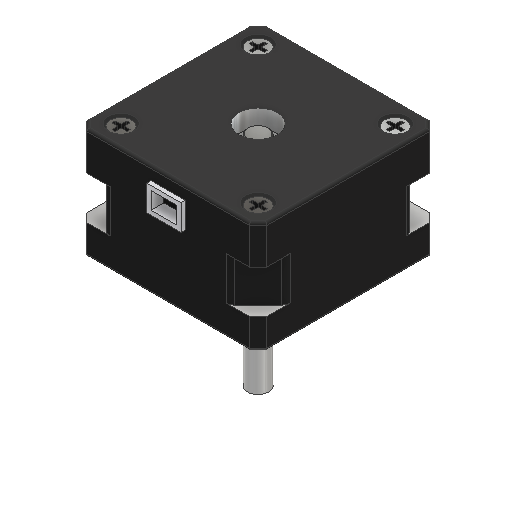
# Autodesk Inventor part: COTS_E3D_NEMA17_Pancake_Stepper_Extruder
Saved by Autodesk Inventor 2026.1 (Build 301233000, 233)
## iProperties
Created: 2016-01-19
Part Number: COTS_E3D_NEMA17_Pancake_Stepper_Extruder
Material: Ogólny
Document SubType Name: Modeling
Designer: Andrzej
Density: 1 g/cm^3
Appearance: Kauczuk - czarny
Mass: 82.3413 g
Surface Area: 122.845 cm^2
Volume: 82.3413 cm^3
Author: Andrzej
Autodesk Inventor part; units mm, degrees
ref_plane "YZ Plane" through (0, 0, 0) normal (1, 0, 0) x (0, 1, 0)
ref_plane "XZ Plane" through (0, 0, 0) normal (0, 1, 0) x (-1, 0, 0)
ref_plane "XY Plane" through (0, 0, 0) normal (0, 0, 1) x (1, 0, 0)
sketch "Szkic1" plane through (0, 0, 0) normal (0, 0, 1) x (1, 0, 0)
  line L0 (-18.7306, 19.0987) -> (23.2694, 19.0987)
  line L1 (23.2694, 19.0987) -> (23.2694, -22.9013)
  line L2 (23.2694, -22.9013) -> (-18.7306, -22.9013)
  line L3 (-18.7306, -22.9013) -> (-18.7306, 19.0987)
  point P0 (0, 0)
  dimension "d0" = 42
  dimension "d1" = 42
  constraints: 8 end point, 2 parallel, 1 horizontal, 1 perpendicular
  measures "d0" distance of L1.end L2.end
  measures "d1" distance of L0.end L1.end
extrude "Wyciągnięcie proste1" add sketch "Szkic1" along normal blind 9
chamfer "Faza1" distance 2 angle 45 4 edges at (23.2694, 19.0987, 4.5) (-18.7306, 19.0987, 4.5) (-18.7306, -22.9013, 4.5) (23.2694, -22.9013, 4.5)
sketch "Szkic2" plane through (0, 0, 0) normal (0, 0, -1) x (-1, 0, 0)
  line L0 (-21.2694, -22.9013) -> (-23.2694, -20.9013) projected
  line L1 (-21.2694, -22.9013) -> (16.7306, -22.9013) projected
  line L2 (18.7306, -20.9013) -> (16.7306, -22.9013) projected
  line L3 (18.7306, -20.9013) -> (18.7306, 17.0987) projected
  line L4 (16.7306, 19.0987) -> (18.7306, 17.0987) projected
  line L5 (16.7306, 19.0987) -> (-21.2694, 19.0987) projected
  line L6 (-23.2694, 17.0987) -> (-21.2694, 19.0987) projected
  line L7 (-23.2694, 17.0987) -> (-23.2694, -20.9013) projected
  line L8 (12.0859, 19.0987) -> (-16.6247, 19.0987)
  line L9 (-23.2694, -16.2567) -> (-16.6247, -22.9013)
  line L10 (12.0859, -22.9013) -> (18.7306, -16.2567)
  line L11 (-23.2694, 12.454) -> (-16.6247, 19.0987)
  line L12 (12.0859, 19.0987) -> (18.7306, 12.454)
  line L13 (-16.6247, 19.0987) -> (12.0859, 19.0987)
  line L14 (-23.2694, 17.0987) -> (-23.2694, -20.9013) projected
  line L15 (-23.2694, 12.454) -> (-23.2694, -16.2567)
  line L16 (-23.2694, -16.2567) -> (-23.2694, 12.454)
  line L17 (-16.6247, -22.9013) -> (12.0859, -22.9013)
  line L18 (-16.6247, -22.9013) -> (12.0859, -22.9013)
  line L19 (18.7306, -16.2567) -> (18.7306, 12.454)
  point P0 (0, 0)
  point P1 (-2.2694, -1.9013)
  dimension "d9" = 21
  dimension "d10" = 42
  dimension "d11" = 21
  dimension "d12" = 25
  dimension "d13" = 25
  dimension "d14" = 25
  dimension "d15" = 25
  constraints: 25 end point, 3 collinear, 2 perpendicular, 1 parallel, 1 point on line
  measures "d9" distance from line of point (-2.269, -1.901) L7
  measures "d10" distance between parallel lines of L3 L7
  measures "d11" distance from line of L5 point (-2.269, -1.901)
  measures "d12" distance from line of L9 point (-2.269, -1.901)
  measures "d13" distance from line of L12 point (-2.269, -1.901)
  measures "d14" distance from line of L11 point (-2.269, -1.901)
  measures "d15" distance from line of L10 point (-2.269, -1.901)
extrude "Wyciągnięcie proste3" add sketch "Szkic2" along normal blind 10 contours L9 L7 L11 L5 L12 L3 L10 L1
sketch "Szkic3" plane through (0, 0, -10) normal (0, 0, -1) x (-1, 0, 0)
  line L0 (-23.2694, -16.2567) -> (-16.6247, -22.9013) projected
  line L1 (-16.6247, -22.9013) -> (12.0859, -22.9013) projected
  line L2 (12.0859, -22.9013) -> (18.7306, -16.2567) projected
  line L3 (18.7306, -16.2567) -> (18.7306, 12.454) projected
  line L4 (18.7306, 12.454) -> (12.0859, 19.0987) projected
  line L5 (12.0859, 19.0987) -> (-16.6247, 19.0987) projected
  line L6 (-16.6247, 19.0987) -> (-23.2694, 12.454) projected
  line L7 (-23.2694, 12.454) -> (-23.2694, -16.2567) projected
  line L8 (-23.2694, 12.454) -> (-16.6247, 19.0987) projected
  line L9 (-16.6247, 19.0987) -> (-21.2694, 19.0987) projected
  line L10 (-23.2694, 17.0987) -> (-21.2694, 19.0987) projected
  line L11 (-23.2694, 17.0987) -> (-23.2694, 12.454) projected
  line L12 (-16.6247, -22.9013) -> (-23.2694, -16.2567) projected
  line L13 (-23.2694, -16.2567) -> (-23.2694, -20.9013) projected
  line L14 (-21.2694, -22.9013) -> (-23.2694, -20.9013) projected
  line L15 (-21.2694, -22.9013) -> (-16.6247, -22.9013) projected
  line L16 (18.7306, -16.2567) -> (12.0859, -22.9013) projected
  line L17 (12.0859, -22.9013) -> (16.7306, -22.9013) projected
  line L18 (18.7306, -20.9013) -> (16.7306, -22.9013) projected
  line L19 (18.7306, -20.9013) -> (18.7306, -16.2567) projected
  line L20 (12.0859, 19.0987) -> (18.7306, 12.454) projected
  line L21 (18.7306, 12.454) -> (18.7306, 17.0987) projected
  line L22 (16.7306, 19.0987) -> (18.7306, 17.0987) projected
  line L23 (16.7306, 19.0987) -> (12.0859, 19.0987) projected
  line L24 (-23.2694, 19.0987) -> (-23.2694, -22.9013)
  line L25 (-23.2694, -22.9013) -> (18.7306, -22.9013)
  line L26 (18.7306, -22.9013) -> (18.7306, 19.0987)
  line L27 (18.7306, 19.0987) -> (-23.2694, 19.0987)
  point P0 (0, 0)
  constraints: 8 end point, 1 perpendicular, 1 point on line
extrude "Wyciągnięcie proste4" add sketch "Szkic3" along normal blind 7 contours L7 L6 L5 L4 L3 L2 L1 L0 | L0 L15 L14 L13 | L11 L10 L9 L6 | L2 L19 L18 L17 | L23 L22 L21 L4
fillet "Zaokrąglenie1" radius 2 8 edges at (-18.7306, 12.454, -5) (-12.0859, 19.0987, -5) (16.6247, 19.0987, -5) (23.2694, 12.454, -5) (-18.7306, -16.2567, -5) (-12.0859, -22.9013, -5) (16.6247, -22.9013, -5) (23.2694, -16.2567, -5)
sketch "Szkic4" plane through (0, 0, 9) normal (0, 0, 1) x (1, 0, 0)
  line L0 (-18.7306, 17.0987) -> (-18.7306, -20.9013) projected
  line L1 (23.2694, -20.9013) -> (23.2694, 17.0987) projected
  line L2 (21.2694, 19.0987) -> (-16.7306, 19.0987) projected
  circle A0 centre (2.2694, -1.9013) radius 4.5
  line L3 (23.2694, 19.0987) -> (-18.7306, 19.0987)
  line L4 (23.2694, -22.9013) -> (-18.7306, -22.9013)
  line L5 (21.2694, -22.9013) -> (-16.7306, -22.9013) projected
  line L6 (-18.7306, -22.9013) -> (-18.7306, 19.0987)
  line L7 (23.2694, 19.0987) -> (23.2694, -22.9013)
  circle A1 centre (-13.7306, 14.0987) radius 2.5
  circle A2 centre (-13.7306, -17.9013) radius 2.5
  circle A3 centre (18.2694, -17.9013) radius 2.5
  circle A4 centre (18.2694, 14.0987) radius 2.5
  circle A5 centre (2.2694, -1.9013) radius 2.5
  circle A6 centre (2.2694, -1.9013) radius 4.25
  circle A7 centre (2.2694, -1.9013) radius 2.75
  point P0 (0, 0)
  dimension "d21" = 42
  dimension "d22" = 21
  dimension "d23" = 21
  dimension "d24" = 9
  dimension "d56" = 5
  dimension "d57" = 5
  dimension "d58" = 5
  dimension "d59" = 5
  dimension "d60" = 5
  dimension "d61" = 5
  dimension "d62" = 5
  dimension "d63" = 5
  dimension "d64" = 5
  dimension "d65" = 5
  dimension "d66" = 5
  dimension "d67" = 5
  dimension "d68" = 5
  dimension "d69" = 8.5
  dimension "d70" = 5.5
  constraints: 8 centre point, 8 coincident, 8 end point, 3 collinear, 1 point on line
  measures "d21" distance between parallel lines of L0 L1
  measures "d22" distance from line of L2 point (2.269, -1.901)
  measures "d23" distance from line of L1 point (2.269, -1.901)
  measures "d24" diameter of A0
  measures "d56" distance from line of L0 point (-13.731, 14.099)
  measures "d57" distance from line of L2 point (-13.731, 14.099)
  measures "d58" distance from line of L2 point (18.269, 14.099)
  measures "d59" distance from line of point (18.269, 14.099) L1
  measures "d60" distance from line of L1 point (18.269, -17.901)
  measures "d61" distance from line of L4 point (18.269, -17.901)
  measures "d62" distance from line of L4 point (-13.731, -17.901)
  measures "d63" distance from line of L0 point (-13.731, -17.901)
  measures "d64" diameter of A1
  measures "d65" diameter of A2
  measures "d66" diameter of A3
  measures "d67" diameter of A4
  measures "d68" diameter of A5
  measures "d69" diameter of A6
  measures "d70" diameter of A7
extrude "Wyciągnięcie proste5" cut sketch "Szkic4" against normal blind 4 contours A0 | A5 | A6 | A7
fillet "Zaokrąglenie2" radius 0.6 16 edges at (23.2694, -1.9013, 9) (2.2694, -22.9013, 9) (-18.7306, -1.9013, 9) (2.2694, 19.0987, 9) (22.2694, -21.9013, 9) (-17.7306, -21.9013, 9) (-17.7306, 18.0987, 9) (22.2694, 18.0987, 9) (23.2694, -1.9013, -17) (22.2694, 18.0987, -17) (2.2694, 19.0987, -17) (-17.7306, 18.0987, -17) (-18.7306, -1.9013, -17) (-17.7306, -21.9013, -17) (2.2694, -22.9013, -17) (22.2694, -21.9013, -17)
sketch "Szkic5" plane through (0, 0, -17) normal (0, 0, -1) x (-1, 0, 0)
  circle A0 centre (-2.2694, -1.9013) radius 4.5 projected
  line L0 (-21.2694, -22.9013) -> (16.7306, -22.9013) projected
  line L1 (16.7306, -22.9013) -> (18.7306, -20.9013) projected
  line L2 (18.7306, -20.9013) -> (18.7306, 17.0987) projected
  line L3 (18.7306, 17.0987) -> (16.7306, 19.0987) projected
  line L4 (16.7306, 19.0987) -> (-21.2694, 19.0987) projected
  line L5 (-21.2694, 19.0987) -> (-23.2694, 17.0987) projected
  line L6 (-23.2694, 17.0987) -> (-23.2694, -20.9013) projected
  line L7 (-23.2694, -20.9013) -> (-21.2694, -22.9013) projected
  line L8 (18.7306, -22.9013) -> (18.7306, 19.0987)
  line L9 (18.7306, 19.0987) -> (-23.2694, 19.0987)
  line L10 (-23.2694, 19.0987) -> (-23.2694, -22.9013)
  line L11 (-23.2694, -22.9013) -> (18.7306, -22.9013)
  circle A1 centre (-2.2694, -1.9013) radius 11
  circle A2 centre (-2.2694, -1.9013) radius 16.25
  circle A3 centre (-2.2694, -1.9013) radius 2.5
  point P0 (0, 0)
  point P1 (13.2306, -17.4013)
  point P2 (13.2306, 13.5987)
  point P3 (-17.7694, 13.5987)
  point P4 (-17.7694, -17.4013)
  dimension "d28" = 42
  dimension "d29" = 5.5
  dimension "d30" = 5.5
  dimension "d31" = 5.5
  dimension "d32" = 5.5
  dimension "d33" = 5.5
  dimension "d34" = 5.5
  dimension "d35" = 5.5
  dimension "d36" = 5.5
  dimension "d37" = 22
  dimension "d38" = 32.5
  dimension "d53" = 5
  dimension "d117" = 21
  dimension "d118" = 21
  constraints: 8 end point, 3 centre point, 1 coincident, 1 collinear, 1 perpendicular, 1 point on line, 1 vertical
  measures "d28" distance between parallel lines of L4 L0
  measures "d29" distance from line of L0 point (13.231, -17.401)
  measures "d30" distance from line of L4 point (13.231, 13.599)
  measures "d31" distance from line of L2 point (13.231, 13.599)
  measures "d32" distance from line of L4 point (-17.769, 13.599)
  measures "d33" distance from line of L6 point (-17.769, 13.599)
  measures "d34" distance from line of L6 point (-17.769, -17.401)
  measures "d35" distance from line of L0 point (-17.769, -17.401)
  measures "d36" distance from line of L2 point (13.231, -17.401)
  measures "d37" diameter of A1
  measures "d38" diameter of A2
  measures "d53" diameter of A3
  measures "d117" distance from line of L0 A1.centre
  measures "d118" distance from line of L2 A0.centre
extrude "Wyciągnięcie proste6" cut sketch "Szkic5" against normal blind 0.3 contours A2
extrude "Wyciągnięcie proste7" add sketch "Szkic5" along normal blind 2 contours A1
chamfer "Faza2" distance 0.5 angle 45 1 edges at (6.7694, -1.9013, -19)
hole "Otwór1" at (-13.2306, -17.4013, -17) at (-13.2306, 13.5987, -17) at (17.7694, 13.5987, -17) at (17.7694, -17.4013, -17) direction (0, 0, 1) diameter 3 depth 5 tip angle 118
extrude "Wyciągnięcie proste8" add sketch "Szkic5" along normal blind 27 contours A3
extrude "Wyciągnięcie proste9" cut sketch "Szkic4" against normal blind 0.5 contours A1 | A2 | A3 | A4
chamfer "Faza3" distance 0.5 angle 45 4 edges at (-16.2306, 14.0987, 9) (15.7694, 14.0987, 9) (15.7694, -17.9013, 9) (-16.2306, -17.9013, 9)
sketch "Szkic6" plane through (2.2694, -1.9013, 5) normal (0, 0, 1) x (1, 0, 0)
  circle A0 centre (0, 0) radius 4.5 projected
  circle A1 centre (0, 0) radius 2.5 projected
  circle A2 centre (0, 0) radius 4.25
  circle A3 centre (0, 0) radius 2.75
  point P0 (-2.2694, 1.9013)
  dimension "d76" = 0.25
  dimension "d77" = 0.25
  constraints: 2 centre point
  measures "d76" radial gap between concentric circles of A0 A2
  measures "d77" radial gap between concentric circles of A1 A3
extrude "Wyciągnięcie proste10" add sketch "Szkic6" along normal blind 2 contours A1
extrude "Wyciągnięcie proste11" cut sketch "Szkic6" against normal blind 0.25
chamfer "Faza4" distance 0.2 angle 45 1 edges at (-0.2306, -1.9013, 7)
sketch "Szkic7" plane through (-13.7306, 14.0987, 8.5) normal (0, 0, 1) x (1, 0, 0)
  circle A0 centre (0, 0) radius 2.5 projected
  circle A1 centre (32, 0) radius 2.5 projected
  circle A2 centre (32, -32) radius 2.5 projected
  circle A3 centre (0, -32) radius 2.5 projected
  line L0 (-0.375, 1.75) -> (0.375, 1.75)
  line L1 (0.375, -1.75) -> (-0.375, -1.75)
  line L2 (1.75, 0.375) -> (1.75, -0.375)
  line L3 (-1.75, -0.375) -> (-1.75, 0.375)
  line L4 (-1.75, 0.375) -> (-0.375, 0.375)
  line L5 (0.375, 0.375) -> (1.75, 0.375)
  line L6 (-0.375, -1.75) -> (-0.375, -0.375)
  line L7 (-0.375, 0.375) -> (-0.375, 1.75)
  line L8 (1.75, -0.375) -> (0.375, -0.375)
  line L9 (-0.375, -0.375) -> (-1.75, -0.375)
  line L10 (0.375, 1.75) -> (0.375, 0.375)
  line L11 (0.375, -0.375) -> (0.375, -1.75)
  line L12 (31.625, 1.75) -> (32.375, 1.75)
  line L13 (32.375, -1.75) -> (31.625, -1.75)
  line L14 (33.75, 0.375) -> (33.75, -0.375)
  line L15 (30.25, -0.375) -> (30.25, 0.375)
  line L16 (30.25, 0.375) -> (31.625, 0.375)
  line L17 (32.375, 0.375) -> (33.75, 0.375)
  line L18 (31.625, -1.75) -> (31.625, -0.375)
  line L19 (31.625, 0.375) -> (31.625, 1.75)
  line L20 (33.75, -0.375) -> (32.375, -0.375)
  line L21 (31.625, -0.375) -> (30.25, -0.375)
  line L22 (32.375, 1.75) -> (32.375, 0.375)
  line L23 (32.375, -0.375) -> (32.375, -1.75)
  line L24 (-0.375, -30.25) -> (0.375, -30.25)
  line L25 (0.375, -33.75) -> (-0.375, -33.75)
  line L26 (1.75, -31.625) -> (1.75, -32.375)
  line L27 (-1.75, -32.375) -> (-1.75, -31.625)
  line L28 (-1.75, -31.625) -> (-0.375, -31.625)
  line L29 (0.375, -31.625) -> (1.75, -31.625)
  line L30 (-0.375, -33.75) -> (-0.375, -32.375)
  line L31 (-0.375, -31.625) -> (-0.375, -30.25)
  line L32 (1.75, -32.375) -> (0.375, -32.375)
  line L33 (-0.375, -32.375) -> (-1.75, -32.375)
  line L34 (0.375, -30.25) -> (0.375, -31.625)
  line L35 (0.375, -32.375) -> (0.375, -33.75)
  line L36 (31.625, -30.25) -> (32.375, -30.25)
  line L37 (32.375, -33.75) -> (31.625, -33.75)
  line L38 (33.75, -31.625) -> (33.75, -32.375)
  line L39 (30.25, -32.375) -> (30.25, -31.625)
  line L40 (30.25, -31.625) -> (31.625, -31.625)
  line L41 (32.375, -31.625) -> (33.75, -31.625)
  line L42 (31.625, -33.75) -> (31.625, -32.375)
  line L43 (31.625, -31.625) -> (31.625, -30.25)
  line L44 (33.75, -32.375) -> (32.375, -32.375)
  line L45 (31.625, -32.375) -> (30.25, -32.375)
  line L46 (32.375, -30.25) -> (32.375, -31.625)
  line L47 (32.375, -32.375) -> (32.375, -33.75)
  point P0 (13.7306, -14.0987)
  dimension "d85" = 0.75
  dimension "d86" = 3.5
  dimension "d88" = 1.75
  dimension "d89" = 3.5
  dimension "d90" = 0.75
  dimension "d91" = 1.75
  dimension "d93" = 0.75
  dimension "d94" = 3.5
  dimension "d95" = 3.5
  dimension "d96" = 0.75
  dimension "d97" = 0.75
  dimension "d98" = 3.5
  dimension "d99" = 3.5
  dimension "d100" = 0.75
  dimension "d101" = 0.75
  dimension "d102" = 3.5
  dimension "d103" = 3.5
  dimension "d104" = 0.75
  constraints: 96 end point, 40 parallel, 16 perpendicular, 12 horizontal
  measures "d85" distance of L1.start L1.end
  measures "d86" distance of L0.end L1.start
  measures "d88" distance from line of L0 A0.centre
  measures "d89" distance of L2.end L3.start
  measures "d90" distance of L2.start L2.end
  measures "d91" distance from line of L3 A0.centre
  measures "d93" distance of L13.start L13.end
  measures "d94" distance of L22.start L13.start
  measures "d95" distance of L14.end L21.end
  measures "d96" distance of L14.start L14.end
  measures "d97" distance of L25.start L25.end
  measures "d98" distance of L34.start L25.start
  measures "d99" distance of L26.end L33.end
  measures "d100" distance of L26.start L26.end
  measures "d101" distance of L37.start L37.end
  measures "d102" distance of L46.start L37.start
  measures "d103" distance of L38.end L45.end
  measures "d104" distance of L38.start L38.end
extrude "Wyciągnięcie proste12" cut sketch "Szkic7" against normal blind 2 contours L0 L10 L5 L2 L8 L11 L1 L6 L9 L3 L4 L7 | L12 L22 L17 L14 L20 L23 L13 L18 L21 L15 L16 L19 | L24 L34 L29 L26 L32 L35 L25 L30 L33 L27 L28 L31 | L36 L46 L41 L38 L44 L47 L37 L42 L45 L39 L40 L43
sketch "Szkic8" plane through (15.7963, -22.9013, -10) normal (0, -1, 0) x (1, 0, 0)
  line L0 (5.4731, -6.4) -> (-32.5269, -6.4) projected
  line L1 (5.4731, 0) -> (5.4731, -6.4) projected
  line L2 (0, 0) -> (5.4731, 0) projected
  line L3 (0, 10) -> (0, 0) projected
  line L4 (5.4731, 10) -> (0, 10) projected
  line L5 (5.4731, 18.4) -> (5.4731, 10) projected
  line L6 (-32.5269, 18.4) -> (5.4731, 18.4) projected
  line L7 (-32.5269, 10) -> (-32.5269, 18.4) projected
  line L8 (-27.0538, 10) -> (-32.5269, 10) projected
  line L9 (-27.0538, 0) -> (-27.0538, 10) projected
  line L10 (-32.5269, 0) -> (-27.0538, 0) projected
  line L11 (-32.5269, 0) -> (-32.5269, -6.4) projected
  line L12 (0, 10) -> (5.4731, 10) projected
  line L13 (-27.0538, 10) -> (0, 10)
  line L14 (-17.5269, 10) -> (-9.5269, 10)
  line L15 (-9.5269, 10) -> (-9.5269, 16)
  line L16 (-9.5269, 16) -> (-17.5269, 16)
  line L17 (-17.5269, 16) -> (-17.5269, 10)
  line L18 (-10.5269, 15) -> (-10.5269, 11)
  line L19 (-10.5269, 11) -> (-16.5269, 11)
  line L20 (-16.5269, 11) -> (-16.5269, 15)
  line L21 (-16.5269, 15) -> (-10.5269, 15)
  point P0 (-15.7963, 10)
  dimension "d107" = 8
  dimension "d108" = 6
  dimension "d109" = 38
  dimension "d110" = 15
  dimension "d111" = 1
  constraints: 18 end point, 4 parallel, 2 horizontal, 2 perpendicular, 1 point on line, 3 other
  measures "d107" distance of L16.end L15.end
  measures "d108" distance of L15.end L14.end
  measures "d109" distance between parallel lines of L5 L7
  measures "d110" distance between parallel lines of L7 L17
  measures "d111" distance between parallel lines of L15 L18
extrude "Wyciągnięcie proste13" add sketch "Szkic8" along normal blind 1 contours L13 L17 L16 L15
extrude "Wyciągnięcie proste14" cut sketch "Szkic8" against normal blind 2 contours L18 L19 L20 L21
equation "\"d13\" = d12"
equation "\"d14\" = d12"
equation "\"d15\" = d12"
equation "\"d22\" = 0.5 * d21"
equation "\"d23\" = 0.5 * d21"
equation "\"d57\" = d56"
equation "\"d58\" = d56"
equation "\"d59\" = d56"
equation "\"d60\" = d56"
equation "\"d61\" = d56"
equation "\"d62\" = d56"
equation "\"d63\" = d56"
equation "\"d30\" = d29"
equation "\"d31\" = d29"
equation "\"d32\" = d29"
equation "\"d33\" = d31"
equation "\"d34\" = d29"
equation "\"d35\" = d29"
equation "\"d36\" = d29"
equation "\"d88\" = 0.5 * d86"
equation "\"d91\" = d88"
equation "\"d110\" = -0.5 * d107 + 0.5 * d109"
equation "\"d87\" = 0.5 * d85"
equation "\"d92\" = d87"
